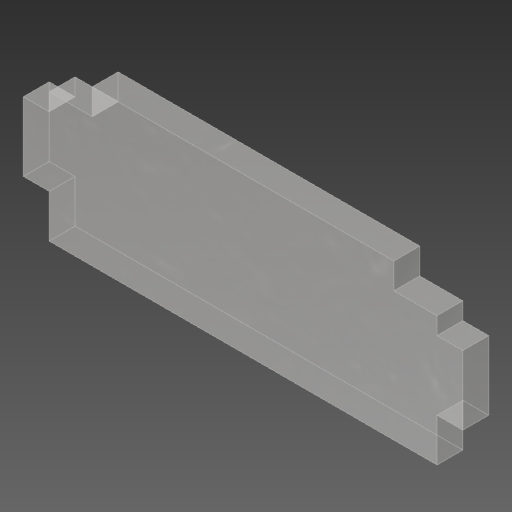
# Autodesk Inventor part: SideFaceTopNM
Saved by Autodesk Inventor 2019 (Build 230136000, 136)
## iProperties
Created: 2019-05-08
Part Number: SideFaceTopNM
Material: Acrylic, Clear
Document SubType Name: Modeling
Designer: super pig
Density: 1.19 g/cm^3
Appearance: Transparent - Clear
Mass: 2.95596 g
Surface Area: 20.7 cm^2
Volume: 2.484 cm^3
Name: Top Face Cover
Author: super pig
Autodesk Inventor part; units mm, degrees
ref_plane "YZ Plane" through (0, 0, 0) normal (1, 0, 0) x (0, 1, 0)
ref_plane "XZ Plane" through (0, 0, 0) normal (0, 1, 0) x (-1, 0, 0)
ref_plane "XY Plane" through (0, 0, 0) normal (0, 0, 1) x (1, 0, 0)
sketch "Sketch1" plane through (0, 0, 0) normal (0, 0, 1) x (1, 0, 0)
  line L0 (5, 0) -> (5, 3) projected
  line L1 (5, 0) -> (40, 0) projected
  line L2 (40, 0) -> (40, 3) projected
  line L3 (5, 3) -> (40, 3) projected
  line L4 (0, 0) -> (5, 0) projected
  line L5 (5, 0) -> (5, 3) projected
  line L6 (0, 3) -> (5, 3) projected
  line L7 (0, 0) -> (0, 3) projected
  line L8 (0, -2) -> (0, 3) projected
  line L9 (0, 3) -> (-3, 3) projected
  line L10 (-3, -2) -> (-3, 3) projected
  line L11 (0, -2) -> (-3, -2) projected
  line L12 (0, -10) -> (-3, -10) projected
  line L13 (0, -10) -> (0, -2) projected
  line L14 (0, -2) -> (-3, -2) projected
  line L15 (-3, -10) -> (-3, -2) projected
  line L16 (0, -15) -> (0, -10) projected
  line L17 (0, -10) -> (-3, -10) projected
  line L18 (-3, -15) -> (-3, -10) projected
  line L19 (0, -15) -> (-3, -15) projected
  line L20 (45, -10) -> (45, -15) projected
  line L21 (45, -15) -> (48, -15) projected
  line L22 (48, -10) -> (48, -15) projected
  line L23 (45, -10) -> (48, -10) projected
  line L24 (45, -2) -> (45, -10) projected
  line L25 (45, -10) -> (48, -10) projected
  line L26 (48, -2) -> (48, -10) projected
  line L27 (45, -2) -> (48, -2) projected
  line L28 (45, 3) -> (45, -2) projected
  line L29 (45, -2) -> (48, -2) projected
  line L30 (48, 3) -> (48, -2) projected
  line L31 (45, 3) -> (48, 3) projected
  line L32 (40, 0) -> (45, 0) projected
  line L33 (45, 0) -> (45, 3) projected
  line L34 (40, 3) -> (45, 3) projected
  line L35 (40, 0) -> (40, 3) projected
  line L36 (0, -15) -> (45, -15)
  constraints: 2 end point, 1 horizontal
extrude "Extrusion1" add sketch "Sketch1" along normal blind 3 contours L0 L3 L2 L1 | L1 L32 L28 L24 L20 L36 L16 L13 L8 L4 | L13 L12 L15 L11 | L27 L26 L23 L24
body "Solid1"
